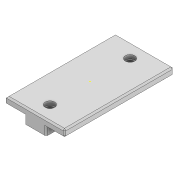
# Autodesk Inventor part: Hanging bracket male
Saved by Autodesk Inventor 2021 (Build 250183000, 183)
## iProperties
Created: 2020-10-29
Part Number: Hanging bracket male
Material: Generic
Document SubType Name: Modeling
Designer: Alfred Brauner
Density: 1 g/cm^3
Appearance: Default
Author: Alfred Brauner
Autodesk Inventor part; units mm, degrees
ref_plane "YZ Plane" through (0, 0, 0) normal (1, 0, 0) x (0, 1, 0)
ref_plane "XZ Plane" through (0, 0, 0) normal (0, 1, 0) x (-1, 0, 0)
ref_plane "XY Plane" through (0, 0, 0) normal (0, 0, 1) x (1, 0, 0)
sketch "Sketch3" plane through (0, 0, 0) normal (0, 0, 1) x (1, 0, 0)
  line L0 (-40, 0) -> (-40, 10)
  line L1 (-40, 10) -> (40, 10)
  line L2 (40, 10) -> (40, 0)
  line L3 (-40, 0) -> (-15, 0)
  line L4 (-15, 0) -> (-15, -10)
  line L5 (-15, -10) -> (15, -10)
  line L6 (15, -10) -> (15, 0)
  line L7 (15, 0) -> (40, 0)
  point P0 (0, 0)
  dimension "d0" = 40
  dimension "d1" = 10
  dimension "d2" = 80
  dimension "d6" = 25
  dimension "d7" = 10
  dimension "d8" = 30
  dimension "d9" = 10
  constraints: 16 end point, 4 perpendicular, 1 horizontal, 1 point on line
  measures "d0" distance of point (0, 0) L0.start
  measures "d1" distance of L0.start L0.end
  measures "d2" distance of L0.end L1.end
  measures "d6" distance of L0.start L3.end
  measures "d7" distance of L3.end L4.end
  measures "d8" distance of L4.end L5.end
  measures "d9" distance of L5.end L6.end
extrude "Extrusion1" add sketch "Sketch3" along normal mid plane 150
sketch "Sketch4" plane through (-40, 10, 75) normal (0, 1, 0) x (1, 0, 0)
  point P0 (40, 75)
chamfer "Chamfer1" distance 2 angle 45 15 edges at (0, 10, 75) (0, 10, -75) (15, -5, 75) (27.5, 0, 75) (40, 0, 0) (27.5, 0, -75) (40, 5, 75) (40, 10, 0) (40, 5, -75) (-15, -5, 75) (-27.5, 0, -75) (-40, 10, 0) (-40, 5, -75) (-40, 0, 0) (-27.5, 0, 75)
sketch "Sketch5" plane through (-38, 10, -73) normal (0, 1, 0) x (1, 0, 0)
  circle A0 centre (38, -18) radius 5.6308
  circle A1 centre (38, -128) radius 5.6351
  line L0 (-2, -148) -> (76, -148) projected
  line L1 (76, 2) -> (0, 2) projected
  line L2 (76, 0) -> (76, -146) projected
  line L3 (78, -146) -> (78, 0) projected
  point P0 (38, -73)
  dimension "d13" = 20
  dimension "d14" = 20
  dimension "d16" = 40
  dimension "d17" = 40
  constraints: 2 centre point
  measures "d13" distance from line of L0 A1.centre
  measures "d14" distance from line of A0.centre L1
  measures "d16" distance from line of L3 A1.centre
  measures "d17" distance from line of L3 A0.centre
hole "Hole1" at (0, 10, -55) at (0, 10, 55) direction (0, -1, 0) diameter 8.5 end through all counterbore diameter 13 counterbore depth 5
body "Solid1"
